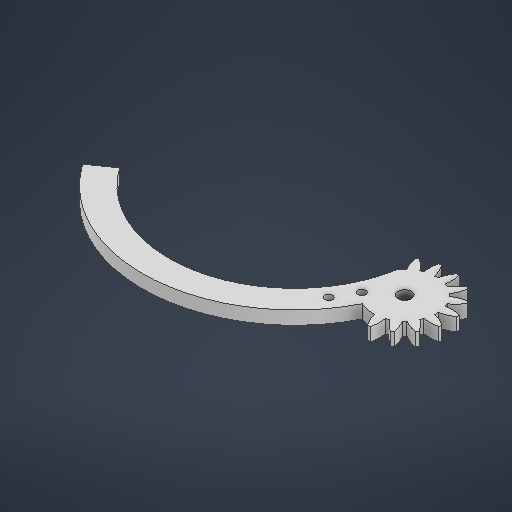
# Autodesk Inventor part: Right_Top_Gripper
Saved by Autodesk Inventor 2026.1 (Build 301233020, 233B)
## iProperties
Created: 2025-10-25
Part Number: Right_Top_Gripper
Material: Generic
Document SubType Name: Modeling
Designer: Garfieldcmix
Density: 1 g/cm^3
Appearance: Default
Author: Garfieldcmix
Autodesk Inventor part; units mm, degrees
ref_plane "YZ Plane" through (0, 0, 0) normal (1, 0, 0) x (0, 1, 0)
ref_plane "XZ Plane" through (0, 0, 0) normal (0, 1, 0) x (-1, 0, 0)
ref_plane "XY Plane" through (0, 0, 0) normal (0, 0, 1) x (1, 0, 0)
derived "Left_Top_Gripper.ipt"
sketch "Sketch1" plane through (0, 0, 0) normal (0, 1, 0) x (-1, 0, 0)
  arc A0 (-44.6354, -16.246) -> (38.9097, -27.2449) centre (0, 0) ccw projected
  line L0 (-44.6354, -16.246) -> (-54.0323, -19.6662) projected
  line L1 (38.9097, -27.2449) -> (47.1012, -32.9806) projected
  arc A1 (-54.0323, -19.6662) -> (47.1012, -32.9806) centre (0, 0) ccw projected
  line L2 (0, -76.3984) -> (0, 12.7331) construction
extrude "Extrusion1" add sketch "Sketch1" along normal blind 5
sketch "Sketch5" plane through (0, 0, 0) normal (0, 1, 0) x (-1, 0, 0)
  arc A0 (-46.8208, -8.0042) -> (-44.6354, -16.246) centre (-56.5705, -15) ccw projected
  line L0 (70.9136, 0) -> (-95.773, 0) construction
  line L1 (-44.6354, -16.246) -> (-54.0323, -19.6662) construction
  arc A1 (-44.6354, -16.246) -> (38.9097, -27.2449) centre (0, 0) ccw construction
  arc A2 (-46.8208, -8.0042) -> (-44.6354, -16.246) centre (0, 0) ccw projected
  circle A3 centre (-56.5705, -15) radius 2.5 projected
extrude "Extrusion3" add sketch "Sketch5" along normal up to surface (5 mm away)
sketch "Sketch11" plane through (0, 5, 0) normal (0, 1, 0) x (0.9914449, 0, 0.1305262)
  circle A0 centre (44.2781, 28.2082) radius 1.5 projected
  circle A1 centre (38.7071, 35.4685) radius 1.5 projected
  point P0 (0, 0)
extrude "Extrusion2" cut sketch "Sketch11" against normal up to surface (5 mm away)
sketch "Sketch12" plane through (-47.1012, 0, -32.9806) normal (0, -1, 0) x (0.819152, 0, 0.5735764)
  line L0 (100.612, -34.0063) -> (103.4791, -36.0138) construction
  arc A0 (104.6268, -30.4084) -> (100.612, -34.0063) centre (111.7881, -42.4382) ccw construction
  line L1 (104.6268, -30.4084) -> (105.4869, -31.0107) construction
  arc A1 (103.4791, -36.0138) -> (105.4869, -31.0107) centre (91.7333, -28.3957) ccw construction
  line L2 (95.2362, -44.7348) -> (102.1191, -34.905) construction
  line L3 (95.2362, -44.7348) -> (103.9046, -36.4367) construction
  arc A2 (84.7774, -50.6181) -> (91.2623, -33.4119) centre (95.2362, -44.7348) ccw construction
  line L4 (105.0221, -37.7895) -> (102.6018, -35.2612)
  line L5 (103.4791, -36.0138) -> (105.4869, -31.0107) construction
  line L6 (100.612, -34.0063) -> (104.6268, -30.4084) construction
  line L7 (102.6018, -35.2612) -> (107.2413, -32.5157) construction
  line L8 (105.0221, -37.7895) -> (107.9674, -33.2742) construction
  line L9 (107.9674, -33.2742) -> (107.2413, -32.5157)
  arc A3 (107.2413, -32.5157) -> (102.6018, -35.2612) centre (111.9181, -45.7114) ccw
  arc A4 (105.0221, -37.7895) -> (107.9674, -33.2742) centre (94.9882, -28.0262) ccw
  point P0 (57.5, 0)
  dimension "d9" = 11.25
  constraints: 11 end point, 7 point on circle, 4 equal length, 2 centre point, 2 equal radius, 2 symmetric about line
  measures "d9" angle of L2 L3
extrude "Extrusion4" add sketch "Sketch12" against normal up to surface (5 mm away)
pattern_circular "Circular Pattern1" count 3 over 45 about axis through (56.5705, 0, -15) along (0, -1, 0) of "Extrusion4"
pattern_circular "Circular Pattern2" count 8 over 157.5 about axis through (56.5705, 0, -15) along (0, 1, 0) of "Extrusion4"
mirror "Mirror1" about plane through (0, 0, 0) normal (0, 0, 1) remove original yes
sketch "Sketch3" plane through (0, 17, 0) normal (0, 1, 0) x (1, 0, 0)
  circle A0 centre (47.5812, 22.1875) radius 1.5 projected
  arc A1 (44.6354, 16.246) -> (36.3871, 30.5324) centre (0, 0) ccw construction
  arc A2 (54.0323, 19.6662) -> (44.0476, 36.9603) centre (0, 0) ccw construction
  line L0 (44.6354, 16.246) -> (54.0323, 19.6662) construction
  line L1 (44.0476, 36.9603) -> (36.3871, 30.5324) construction
  line L2 (43.0496, 20.0744) -> (52.1127, 24.3006) construction
  line L3 (38.9097, 27.2449) -> (47.1012, 32.9806) construction
  circle A3 centre (43.0055, 30.1128) radius 1.5 projected
sketch "Sketch6" plane through (0, 0, 0) normal (0, 1, 0) x (-1, 0, 0)
  arc A0 (-46.8208, -8.0042) -> (-51.3777, -25.8182) centre (-56.5705, -15) ccw construction
  line L0 (-56.5705, -15) -> (-56.5705, -3) construction
  line L1 (-54.8205, -3.1283) -> (-58.3205, -3.1283) projected
  line L2 (-58.3205, -3.1283) -> (-57.0955, 2.1217) construction
  line L3 (-54.8205, -3.1283) -> (-56.0455, 2.1217) construction
  line L4 (-56.0455, 2.1217) -> (-57.0955, 2.1217) projected
  arc A1 (-54.8205, -3.1283) -> (-56.0455, 2.1217) centre (-68.8117, -3.625) ccw projected
  arc A2 (-57.0955, 2.1217) -> (-58.3205, -3.1283) centre (-44.3294, -3.625) ccw projected
  point P0 (0, 0)
body "Solid2"
